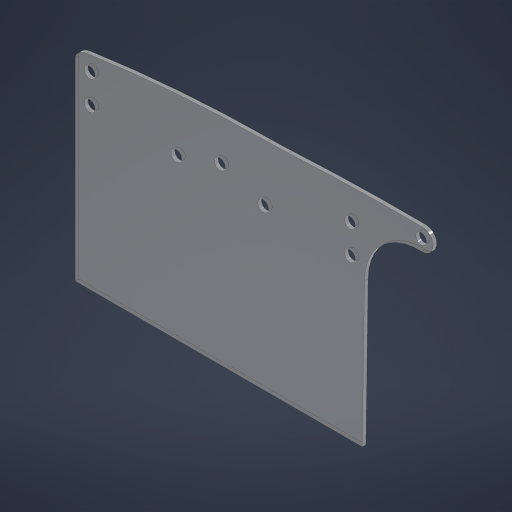
# Autodesk Inventor part: wings
Saved by Autodesk Inventor 2024 (Build 280153000, 153)
## iProperties
Created: 2023-11-18
Part Number: wings
Material: Polycarbonate, Clear
Document SubType Name: Modeling
Designer: macbook
Density: 1.2 g/cm^3
Appearance: Polycarbonate - Clear(1)
Author: macbook
Autodesk Inventor part; units mm, degrees
ref_plane "YZ Plane" through (0, 0, 0) normal (1, 0, 0) x (0, 1, 0)
ref_plane "XZ Plane" through (0, 0, 0) normal (0, 1, 0) x (-1, 0, 0)
ref_plane "XY Plane" through (0, 0, 0) normal (0, 0, 1) x (1, 0, 0)
sketch "Sketch1" plane through (0, 0, 0) normal (0, 0, 1) x (1, 0, 0)
  line L0 (127, 63.5) -> (127, 57.15)
  line L1 (127, 57.15) -> (127, 31.75)
  line L2 (127, 31.75) -> (152.4, 31.75)
  line L3 (0, 60.325) -> (0, 63.5)
  line L4 (0, 63.5) -> (0, 57.15)
  arc A0 (152.4, 57.15) -> (127, 31.75) centre (152.4, 31.75) ccw construction
  line L5 (127, 63.5) -> (152.4, 63.5) construction
  line L6 (152.4, 57.15) -> (152.4, 63.5) construction
  arc A1 (152.4, 57.15) -> (152.4, 63.5) centre (152.4, 60.325) ccw construction
  line L7 (127, 63.5) -> (88.9, 63.5) construction
  line L8 (0, 57.15) -> (1.3137, 57.15)
  line L9 (3.175, 57.15) -> (3.175, 53.975)
  arc A2 (3.175, 57.15) -> (0, 53.975) centre (3.175, 53.975) ccw
  arc A3 (84.3846, 63.4825) -> (4.9889, 57.4173) centre (88.9, -518.3187) ccw
  arc A4 (4.9889, 57.4173) -> (0.7473, 55.0582) centre (5.9749, 50.6519) ccw
  arc A5 (0.7473, 55.0582) -> (0, 53.0119) centre (3.175, 53.0119) ccw
  circle A6 centre (152.4, 60.325) radius 4.7625
  arc A7 (152.1428, 55.5695) -> (127, 31.75) centre (150.8543, 31.75) ccw
  line L10 (127, 60.325) -> (152.4, 60.325) construction
  arc A8 (152.4, 65.0875) -> (93.6534, 63.766) centre (144.3966, -885.5701) ccw
  arc A9 (84.3846, 63.4825) -> (93.6534, 63.766) centre (82.8076, 266.6764) ccw
  line L11 (0, 57.15) -> (0, 31.75)
  line L12 (0, 31.75) -> (0, -31.75)
  line L13 (127, 31.75) -> (126.031, -31.75)
  line L14 (126.031, -31.75) -> (0, -31.75)
  point P0 (127, 44.45)
  point P1 (0, 53.0119)
  dimension "d15" = 6.35
  dimension "d23" = 25.4
  dimension "d24" = 25.4
  dimension "d25" = 6.35
  dimension "d27" = 0
  dimension "d28" = 38.1
  dimension "d29" = 3.175
  dimension "d31" = 3.175
  dimension "d39" = 9.525
  dimension "d40" = 203.2
  dimension "d41" = 25.4
  dimension "d42" = 63.5
  constraints: 30 end point, 24 point on circle, 10 centre point, 6 tangent, 5 horizontal, 3 coincident, 3 midpoint, 3 point on line, 1 perpendicular, 1 vertical
  measures "d15" distance of L0.start L0.end
  measures "d23" distance of L0.end L1.end
  measures "d24" distance of L1.end L2.end
  measures "d25" distance of L3.end L4.end
  measures "d27" distance of L5.end L6.end
  measures "d28" distance of L0.start L7.end
  measures "d29" distance of L9.start L9.end
  measures "d31" radius of A5
  measures "d39" diameter of A6
  measures "d40" radius of A9
  measures "d41" distance of L4.end L11.end
  measures "d42" distance of L11.end L12.end
extrude "Extrusion1" add sketch "Sketch1" along normal blind 1.5875 contours A4 A3 A9 A8 A6 A7 L13 L14 L12 L11 A5 | A6
sketch "Sketch2" plane through (0, 0, 1.5875) normal (0, 0, 1) x (1, 0, 0)
  line L0 (127, 63.5) -> (0, 63.5) projected
  line L1 (0, 63.5) -> (0, 50.8)
  line L2 (0, 63.5) -> (0, 0) projected
  line L3 (0, 50.8) -> (6.35, 50.8)
  line L4 (6.35, 50.8) -> (6.35, 38.1)
  line L5 (6.35, 50.8) -> (120.65, 50.8)
  line L6 (120.65, 50.8) -> (120.65, 38.1)
  line L7 (63.5, 50.8) -> (63.5, 44.45)
  line L8 (127, 63.5) -> (127, 60.325)
  line L9 (127, 60.325) -> (151.892, 60.325)
  line L10 (120.65, 38.1) -> (82.55, 38.1)
  line L11 (6.35, 38.1) -> (44.45, 38.1)
  point P0 (0, 60.325)
  point P1 (3.175, 63.5)
  dimension "d4" = 12.7
  dimension "d5" = 6.35
  dimension "d6" = 12.7
  dimension "d7" = 114.3
  dimension "d32" = 3.175
  dimension "d33" = 24.892
  dimension "d34" = 38.1
  dimension "d35" = 38.1
  constraints: 20 end point, 8 coincident, 4 horizontal, 2 perpendicular, 2 vertical, 1 midpoint, 1 parallel, 1 point on line
  measures "d4" distance of L0.end L1.end
  measures "d5" distance of L1.end L3.end
  measures "d6" distance of L3.end L4.end
  measures "d7" distance of L3.end L5.end
  measures "d32" distance of L0.start L8.end
  measures "d33" distance of L8.end L9.end
  measures "d34" distance of L10.start L10.end
  measures "d35" distance of L11.start L11.end
hole "Hole1" at (6.35, 38.1, 1.5875) at (6.35, 50.8, 1.5875) at (120.65, 38.1, 1.5875) at (120.65, 50.8, 1.5875) at (63.5, 44.45, 1.5875) at (151.892, 60.325, 1.5875) at (44.45, 38.1, 1.5875) at (82.55, 38.1, 1.5875) direction (0, 0, -1) diameter 4.7625 end through all
sketch "Sketch3" plane through (0, 0, 1.5875) normal (0, 0, 1) x (1, 0, 0)
  line L0 (0, 0) -> (0, 31.75)
  line L1 (0, 53.0119) -> (0, 3.175) projected
  line L2 (127, 3.175) -> (127, 31.75) projected
  line L3 (0, 31.75) -> (127, 31.75)
  dimension "d36" = 31.75
  constraints: 4 end point, 1 point on line
  measures "d36" distance of L0.start L0.end
feature "Bend Part1" [suppressed]
body "Solid1"
